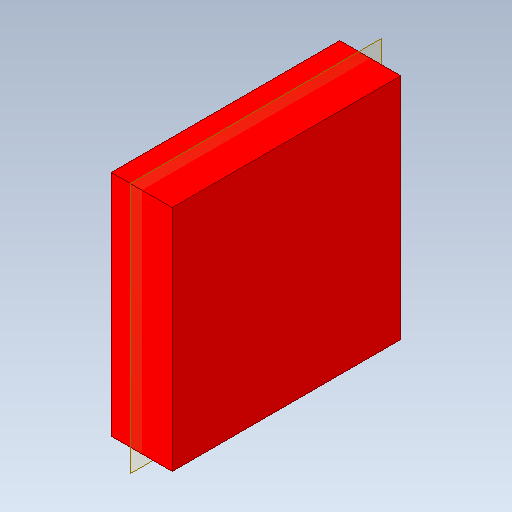
# Autodesk Inventor part: BlockedZone
Saved by Autodesk Inventor 2021 (Build 250183000, 183)
## iProperties
Created: 2019-04-14
Part Number: BlockedZone
Material: Generic
Document SubType Name: Modeling
Designer: CASE-SMALL2
Density: 1 g/cm^3
Appearance: Default
Author: CASE-SMALL2
Autodesk Inventor part; units mm, degrees
ref_plane "YZ Plane" through (0, 0, 0) normal (1, 0, 0) x (0, 1, 0)
ref_plane "XZ Plane" through (0, 0, 0) normal (0, 1, 0) x (-1, 0, 0)
ref_plane "XY Plane" through (0, 0, 0) normal (0, 0, 1) x (1, 0, 0)
sketch "Sketch1" plane through (0, 0, 0) normal (0, 0, 1) x (1, 0, 0)
  point P0 (0, 0)
sketch "Sketch2" plane through (0, 0, 0) normal (0, 0, 1) x (1, 0, 0)
  line L0 (-40, -150) -> (40, -150)
  line L1 (40, -150) -> (40, 150)
  line L2 (40, 150) -> (-40, 150)
  line L3 (-40, 150) -> (-40, -150)
  line L4 (-40, -150) -> (40, 150) construction
  line L5 (40, -150) -> (-40, 150) construction
  point P0 (0, 0)
  dimension "d0" = 300
  dimension "d1" = 80
  constraints: 12 end point, 2 midpoint, 2 parallel, 1 horizontal, 1 perpendicular
  measures "d0" distance of L0.end L1.end
  measures "d1" distance of L1.end L2.end
extrude "Extrusion1" add sketch "Sketch2" along normal blind 300
ref_plane "Work Plane1" through (0, -150, 0) normal (1, 0, 0) x (0, 0, -1)
body "Solid1"
